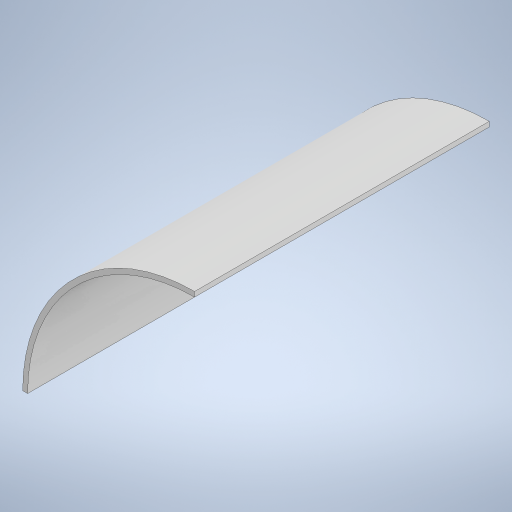
# Autodesk Inventor part: Electronics Door
Saved by Autodesk Inventor 2024 (Build 280153000, 153)
## iProperties
Created: 2024-04-23
Part Number: Electronics Door
Material: Generic
Document SubType Name: Modeling
Designer: auror
Density: 1 g/cm^3
Appearance: Default
Author: auror
Autodesk Inventor part; units mm, degrees
ref_plane "YZ Plane" through (0, 0, 0) normal (1, 0, 0) x (0, 1, 0)
ref_plane "XZ Plane" through (0, 0, 0) normal (0, 1, 0) x (-1, 0, 0)
ref_plane "XY Plane" through (0, 0, 0) normal (0, 0, 1) x (1, 0, 0)
sketch "Sketch1" plane through (0, 0, 0) normal (0, 0, 1) x (1, 0, 0)
  arc A0 (0, 34) -> (-34, 0) centre (0, 0) ccw
  arc A1 (0, 35) -> (-35, 0) centre (0, 0) ccw
  line L0 (-52.4518, 0) -> (56.8215, 0) construction
  line L1 (0, 39.5237) -> (0, -43.4686) construction
  line L2 (-35, 0) -> (-34, 0)
  line L3 (0, 35) -> (0, 34)
  dimension "d0" = 68
  dimension "d1" = 70
  constraints: 8 end point, 4 point on circle, 4 point on line, 2 centre point, 2 coincident, 2 horizontal, 1 collinear, 1 vertical
  measures "d0" diameter of A0
  measures "d1" diameter of A1
extrude "Extrusion1" add sketch "Sketch1" along normal blind 60
body "Solid1"
